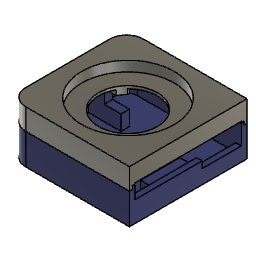
TouchKey-Case (Autodesk Fusion 360 design; units mm, degrees)
Autodesk Fusion 360 part; units mm, degrees
sketch "Sketch2" plane through (0, 0, 0) normal (0, 0, 1) x (1, 0, 0)
  line L0 (3, 21) -> (21.5, 21)
  line L1 (21.5, 21) -> (21.5, 0)
  line L2 (21.5, 0) -> (3, 0)
  line L3 (0, 3) -> (0, 18)
  line L4 (20.5, 20) -> (3, 20)
  line L5 (1, 18) -> (1, 3)
  line L6 (3, 1) -> (20.5, 1)
  line L7 (20.5, 1) -> (20.5, 20)
  line L8 (20.5, 20) -> (21.5, 20)
  line L9 (20.5, 1) -> (21.5, 1)
  line L10 (20.5, 13) -> (21.5, 13)
  line L11 (20.5, 5) -> (18.5, 5)
  line L12 (18.5, 5) -> (18.5, 12)
  line L13 (18.5, 12) -> (20.5, 12)
  line L14 (20.5, 12) -> (20.5, 5)
  line L15 (1, 6.5) -> (4, 6.5)
  line L16 (4, 6.5) -> (4, 8)
  line L17 (4, 8) -> (1, 8)
  line L18 (1, 8) -> (1, 6.5)
  line L19 (1, 14.5) -> (4, 14.5)
  line L20 (4, 14.5) -> (4, 13)
  line L21 (4, 13) -> (1, 13)
  line L22 (1, 13) -> (1, 14.5)
  line L23 (4, 8) -> (7, 8)
  line L24 (7, 8) -> (7, 6.5)
  line L25 (7, 6.5) -> (4, 6.5)
  line L26 (4, 6.5) -> (4, 8)
  line L27 (4, 14.5) -> (7, 14.5)
  line L28 (7, 14.5) -> (7, 13)
  line L29 (7, 13) -> (4, 13)
  line L30 (4, 13) -> (4, 14.5)
  arc A0 (3, 20) -> (1, 18) centre (3, 18) ccw
  arc A1 (3, 21) -> (0, 18) centre (3, 18) ccw
  arc A2 (1, 3) -> (3, 1) centre (3, 3) ccw
  arc A3 (0, 3) -> (3, 0) centre (3, 3) ccw
  line L31 (21.5, 0.5) -> (3, 0.5)
  arc A4 (0.5, 3) -> (3, 0.5) centre (3, 3) ccw
  line L32 (0.5, 3) -> (0.5, 18)
  arc A5 (3, 20.5) -> (0.5, 18) centre (3, 18) ccw
  line L33 (3, 20.5) -> (21.5, 20.5)
  line L34 (21.5, 10.5) -> (0, 10.5) construction
  circle A6 centre (10.75, 10.5) radius 8.25
  circle A7 centre (10.75, 10.5) radius 5.25
  point P0 (0, 21)
  dimension "d1" = 21.5
  dimension "d2" = 21
  dimension "d3" = 12
  dimension "d4" = 2
  dimension "d5" = 7
  dimension "d6" = 3
  dimension "d7" = 1.5
  dimension "d8" = 3
  dimension "d9" = 5.5
  dimension "d10" = 5.5
  dimension "d11" = 2
  dimension "d12" = 3
  dimension "d13" = 2
  dimension "d14" = 3
  dimension "d23" = 0.5
  dimension "d28" = 16.5
  dimension "d29" = 10.5
  constraint horizontal L0
  constraint vertical L1
  constraint horizontal L2
  constraint vertical L3
  constraint horizontal L4
  constraint vertical L5
  constraint horizontal L6
  constraint vertical L7
  constraint coincident L1 L8.end
  constraint perpendicular L1 L8
  constraint coincident L1 L9.end
  constraint perpendicular L1 L9
  constraint perpendicular L7 L10
  constraint coincident L7 L10.start
  constraint coincident L1 L10.end
  constraint horizontal L11
  constraint vertical L12
  constraint horizontal L13
  constraint vertical L14
  constraint coincident L7 L11.start
  constraint horizontal L15
  constraint vertical L16
  constraint horizontal L17
  constraint vertical L18
  constraint coincident L5 L15.start
  constraint horizontal L19
  constraint vertical L20
  constraint horizontal L21
  constraint vertical L22
  constraint coincident L5 L19.start
  constraint horizontal L23
  constraint vertical L24
  constraint horizontal L25
  constraint vertical L26
  constraint horizontal L27
  constraint vertical L28
  constraint horizontal L29
  constraint vertical L30
  constraint tangent L4 A0
  constraint tangent L5 A0
  constraint coincident P0 L0
  constraint coincident P0 L3
  constraint tangent L0 A1
  constraint tangent L3 A1
  constraint tangent L5 A2
  constraint tangent L6 A2
  constraint coincident origin L2
  constraint coincident origin L3
  constraint tangent L2 A3
  constraint tangent L3 A3
  constraint midpoint L3 L34.end
  constraint midpoint L34 A6.centre
  constraint concentric A6 A7
  measures "d1" distance of P0 L0.end
  measures "d2" distance of P0 origin
  measures "d3" distance of L6 L10
  measures "d4" distance of L11.start L11.end
  measures "d5" distance of L11.start L13.end
  measures "d6" distance of L15.start L15.end
  measures "d7" distance of L15.start L17.end
  measures "d8" distance of L19.start L19.end
  measures "d9" distance of L4 L19
  measures "d10" distance of L6 L15
  measures "d11" radius of A0
  measures "d12" radius of A1
  measures "d13" radius of A2
  measures "d14" radius of A3
  measures "d28" diameter of A6
  measures "d29" diameter of A7
extrude "Extrude1" add sketch "Sketch2" along normal blind 5 contours L1 L4 L5 L6 L8 L9 L18 L22 A0 A2 L31 A4 L32 A5 L33 | L5 L19 L21 L22 A6 | L19 L20 L21 L30 A6 | L5 L15 L17 L18 A6 | L15 L16 L17 L26 A6 makes body 1
extrude "Extrude2" add sketch "Sketch2" against normal blind 1 bodies 1
extrude "Extrude3" add sketch "Sketch2" along normal blind 2.7 contours L1 L7 L9 L10 L14 | L20 L27 L28 L29 L30 A7 | L16 L23 L24 L25 L26 A7 | L28 L29 A7 | L23 L24 A7 bodies 1
extrude "Extrude4" add sketch "Sketch2" along normal blind 2.2 contours L7 L11 L12 L13 L14 A6 | L12 L13 A6 bodies 1
extrude "Extrude5" add sketch "Sketch2" along normal blind 4.5 contours L0 L1 L2 L3 A1 A3 L31 A4 L32 A5 L33 bodies 1
extrude "Extrude6" add sketch "Sketch2" along normal blind 1.5 contours L1 L7 L8 L10 bodies 1
ref_plane "WorkPlane1" through (10.3898, 10.5, 6) normal (0, 0, 1) x (1, 0, 0)
extrude "Extrude7" add sketch "Sketch2" along normal blind 2.3 from surface at 6 separate body contours L0 L1 L2 L3 A1 A3 L31 A4 L32 A5 L33 | L1 L4 L5 L6 L8 L9 L18 L22 A0 A2 L31 A4 L32 A5 L33 | L1 L7 L8 L10 | L1 L7 L9 L10 L14 | L4 L5 L7 L13 L19 A0 A6 | L5 L6 L7 L11 L12 L15 A2 A6 | L7 L11 L12 L13 L14 A6 | L5 L19 L21 L22 A6 | L5 L17 L21 A6 | L5 L15 L17 L18 A6 makes body 2
extrude "Extrude8" add sketch "Sketch2" along normal blind 0.5 from surface at 6 separate body contours L12 L13 A6 | L12 L13 L15 L19 L24 L25 L27 L28 A6 A7 | L19 L20 L21 L30 A6 | L20 L27 L28 L29 L30 A7 | L17 L21 L23 L29 A6 A7 | L15 L16 L17 L26 A6 | L16 L23 L24 L25 L26 A7 makes body 3
combine "Combine1" operation add target body 2 tool bodies 3
extrude "Extrude9" add sketch "Sketch2" against normal blind 0.9 from surface at 6 separate body contours L1 L4 L5 L6 L8 L9 L18 L22 A0 A2 L31 A4 L32 A5 L33 makes body 4
extrude "Extrude10" add sketch "Sketch2" against normal blind 1.5 from surface at 6 contours L0 L1 L2 L3 A1 A3 L31 A4 L32 A5 L33 bodies 2 4
extrude "Extrude11" add sketch "Sketch2" against normal blind 0.7 from surface at 6 contours L1 L7 L8 L10 | L1 L7 L9 L10 L14 bodies 2
extrude "Extrude12" add sketch "Sketch2" against normal blind 0.9 from surface at 6 separate body contours L5 L19 L21 L22 A6 | L19 L20 L21 L30 A6 | L5 L15 L17 L18 A6 | L20 L27 L28 L29 L30 A7 | L15 L16 L17 L26 A6 | L16 L23 L24 L25 L26 A7 makes body 5 at (4, 14, 6) makes body 6 at (2.7112, 7.5, 6)
combine "Combine2" operation add target body 2 tool bodies 5 6
named bodies: "Lower shell", "Upper shell"
